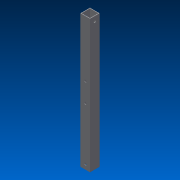
# Autodesk Inventor part: BAseBAr
Saved by Autodesk Inventor 2013 (Build 170138000, 138)
## iProperties
Created: 2013-07-20
Part Number: BAseBAr
Material: Aluminum 6061
Document SubType Name: Modeling
Designer: robotics
Density: 1 g/cm^3
Author: robotics
Autodesk Inventor part; units mm, degrees
ref_plane "YZ Plane" through (0, 0, 0) normal (1, 0, 0) x (0, 1, 0)
ref_plane "XZ Plane" through (0, 0, 0) normal (0, 1, 0) x (-1, 0, 0)
ref_plane "XY Plane" through (0, 0, 0) normal (0, 0, 1) x (1, 0, 0)
sketch "Sketch1" plane through (0, 0, 0) normal (0, 1, 0) x (-1, 0, 0)
  line L0 (-12.7, -12.7) -> (12.7, -12.7)
  line L1 (12.7, -12.7) -> (12.7, 12.7)
  line L2 (12.7, 12.7) -> (-12.7, 12.7)
  line L3 (-12.7, 12.7) -> (-12.7, -12.7)
  line L4 (-12.7, -12.7) -> (12.7, 12.7) construction
  line L5 (12.7, -12.7) -> (-12.7, 12.7) construction
  line L6 (-10.9728, -10.9728) -> (10.9728, -10.9728)
  line L7 (10.9728, -10.9728) -> (10.9728, 10.9728)
  line L8 (10.9728, 10.9728) -> (-10.9728, 10.9728)
  line L9 (-10.9728, 10.9728) -> (-10.9728, -10.9728)
  line L10 (-10.9728, -10.9728) -> (10.9728, 10.9728) construction
  line L11 (10.9728, -10.9728) -> (-10.9728, 10.9728) construction
  point P0 (0, 0)
  dimension "d0" = 25.4
  dimension "d2" = 25.4
  dimension "d3" = 1.7272
  dimension "d4" = 1.7272
  constraints: 24 end point, 4 midpoint, 4 parallel, 2 horizontal, 2 perpendicular
  measures "d0" distance of L1.end L2.end
  measures "d2" distance of L2.end L0.start
  measures "d3" distance between parallel lines of L8 L2
  measures "d4" distance between parallel lines of L1 L7
extrude "Extrusion1" add sketch "Sketch1" along normal blind 352.425
sketch "Sketch2" plane through (12.7, 0, 12.7) normal (1, 0, 0) x (0, 0, -1)
  line L0 (0, 352.425) -> (25.4, 352.425) projected
  line L1 (0, 0) -> (0, 352.425) projected
  point P0 (12.7, 0)
  point P1 (12.7, 339.725)
  dimension "d7" = 12.7
  dimension "d8" = 12.7
  measures "d7" distance from line of L0 point (12.7, 339.725)
  measures "d8" distance from line of point (12.7, 339.725) L1
hole "Hole1" at (12.7, 339.725, 0) direction (-1, 0, 0) diameter 6.35 end through all
sketch "Sketch4" plane through (-12.7, 0, 12.7) normal (0, 0, 1) x (1, 0, 0)
  line L0 (0, 0) -> (25.4, 0) projected
  line L1 (25.4, 0) -> (25.4, 352.425) projected
  point P0 (12.7, 0)
  point P1 (12.7, 12.7)
  dimension "d25" = 12.7
  dimension "d26" = 12.7
  measures "d25" distance from line of L1 point (12.7, 12.7)
  measures "d26" distance from line of L0 point (12.7, 12.7)
hole "Hole3" at (0, 12.7, 12.7) direction (0, 0, -1) diameter 6.35 end through all
sketch "Sketch5" plane through (12.7, 0, -12.7) normal (0, 0, -1) x (-1, 0, 0)
  line L0 (0, 0) -> (25.4, 0) projected
  line L1 (25.4, 0) -> (25.4, 352.425) projected
  line L2 (0, 352.425) -> (25.4, 352.425) projected
  point P0 (12.7, 0)
  point P1 (12.7, 203.2)
  point P2 (12.7, 152.4)
  dimension "d34" = 50.8
  dimension "d36" = 152.4
  dimension "d38" = 149.225
  dimension "d39" = 352.425
  dimension "d40" = 12.7
  dimension "d41" = 12.7
  measures "d34" distance of point (12.7, 152.4) point (12.7, 203.2)
  measures "d36" distance from line of L0 point (12.7, 152.4)
  measures "d38" distance from line of point (12.7, 203.2) L2
  measures "d39" distance of L0.end L1.end
  measures "d40" distance from line of L1 point (12.7, 152.4)
  measures "d41" distance from line of L1 point (12.7, 203.2)
hole "Hole4" at (0, 203.2, -12.7) at (0, 152.4, -12.7) direction (0, 0, 1) diameter 6.35 end through all
body "Solid1"
